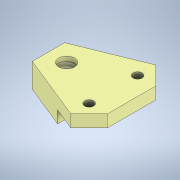
# Autodesk Inventor part: rollertriangle(v3)
Saved by Autodesk Inventor 2022 (Build 260153000, 153)
## iProperties
Created: 2022-11-07
Part Number: rollertriangle(v3)
Material: Generic
Document SubType Name: Modeling
Designer: matia
Density: 1 g/cm^3
Appearance: Default
Author: matia
Autodesk Inventor part; units mm, degrees
ref_plane "YZ Plane" through (0, 0, 0) normal (1, 0, 0) x (0, 1, 0)
ref_plane "XZ Plane" through (0, 0, 0) normal (0, 1, 0) x (-1, 0, 0)
ref_plane "XY Plane" through (0, 0, 0) normal (0, 0, 1) x (1, 0, 0)
sketch "Sketch1" plane through (0, 0, 0) normal (0, 1, 0) x (-1, 0, 0)
  circle A0 centre (0, 0) radius 1.5875
  line L0 (0, 0) -> (0, -7.62)
  circle A1 centre (0, -7.62) radius 1.5875
  line L1 (-14.0081, -3.81) -> (-6.6675, -3.81)
  circle A2 centre (7.3406, -3.81) radius 1.5875
  line L2 (8.9281, -3.81) -> (10.1981, -3.81)
  line L3 (10.1981, -3.81) -> (10.1981, -6.35)
  line L4 (10.1981, -6.35) -> (10.1981, -1.27)
  line L5 (0, 1.5875) -> (0, 2.8575)
  line L6 (-1.5875, 0) -> (-2.8575, 0)
  line L7 (0, -9.2075) -> (0, -10.4775)
  line L8 (-1.5875, -7.62) -> (-2.8575, -7.62)
  line L9 (-2.8575, -7.62) -> (-2.8575, 0)
  line L10 (0, 2.8575) -> (-2.8575, 0)
  line L11 (0, 2.8575) -> (10.1981, -1.27)
  line L12 (10.1981, -6.35) -> (0, -10.4775)
  line L13 (-2.8575, -7.62) -> (0, -10.4775)
  line L14 (-2.8575, -3.81) -> (0, -3.81)
  line L15 (3.4925, -3.81) -> (3.4925, -9.064)
  line L16 (3.4925, -3.81) -> (3.4925, 1.444)
  dimension "d4" = 3.175
  dimension "d0" = 3.175
  dimension "d1" = 7.62
  dimension "d2" = 3.175
  dimension "d3" = 7.3406
  dimension "d5" = 1.27
  dimension "d6" = 2.54
  dimension "d7" = 5.08
  dimension "d8" = 1.27
  dimension "d9" = 1.27
  dimension "d10" = 1.27
  dimension "d11" = 1.27
  dimension "d12" = 6.35
  constraints: 34 end point, 5 horizontal, 5 point on line, 4 perpendicular, 4 point on circle, 3 vertical, 2 centre point, 2 coincident, 2 midpoint, 1 horizontal alignment, 2 other
  measures "d0" diameter of A0
  measures "d1" distance of L0.start L0.end
  measures "d2" diameter of A1
  measures "d3" distance of L1.start L1.end
  measures "d5" distance of L2.start L2.end
  measures "d6" distance of L2.end L3.end
  measures "d7" distance of L3.end L4.end
  measures "d8" distance of L5.start L5.end
  measures "d9" distance of L6.start L6.end
  measures "d10" distance of L7.start L7.end
  measures "d11" distance of L8.start L8.end
  measures "d12" distance of L14.start L15.start
extrude "Extrusion1" add sketch "Sketch1" along normal blind 1.905 contours L11 L4 L3 L12 L15 L16
extrude "Extrusion2" add sketch "Sketch1" along normal blind 1.905 contours A0 | A0 L5 L11 L16 L15 L12 L7 A1 L0 | A0 L6 L10 L5 | L0 L14 L9 L6 A0 | L0 A1 L8 L9 L14 | A1 | A1 L7 L13 L8 | A2
extrude "Extrusion3" add sketch "Sketch1" against normal blind 1.905 contours L11 L4 L3 L12 L15 L16 | A2
hole "Hole1" at (0, 0, -7.62) direction (0, 1, 0) diameter 1.4249 depth 5.6896 thread size "1-64 UNC" class "2B" standard "ANSI Unified Screw Threads"
hole "Hole2" at (0, 0, 0) direction (0, 1, 0) diameter 1.4249 depth 5.6896 thread size "1-64 UNC" class "2B" standard "ANSI Unified Screw Threads"
sketch "Sketch2" plane through (0, -1.905, 0) normal (0, -1, 0) x (1, 0, 0)
  line L0 (-10.1981, -6.35) -> (-10.1981, -1.27) projected
  line L1 (-10.1981, -3.81) -> (-7.3406, -3.81)
  circle A0 centre (-7.3406, -3.81) radius 1.5875
  point P0 (0, 0)
  dimension "d33" = 2.8575
  dimension "d34" = 3.175
  constraints: 2 end point, 1 centre point, 1 coincident, 1 horizontal, 1 midpoint
  measures "d33" distance of L1.start L1.end
  measures "d34" diameter of A0
hole "Hole3" at (-7.3406, -1.905, -3.81) direction (0, 1, 0) diameter 2.4867 depth 9.525 thread size "5-40 UNC" class "2B" standard "ANSI Unified Screw Threads"
equation "\"d36\" = d0"
body "Solid1"
